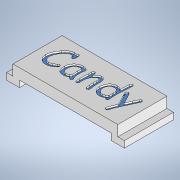
# Autodesk Inventor part: Крышка аккумулятора
Saved by Autodesk Inventor 2020 (Build 240168000, 168)
## iProperties
Created: 2021-04-26
Part Number: Крышка аккумулятора
Material: Типовые
Document SubType Name: Обычные детали
Designer: Антон
Density: 1 g/cm^3
Appearance: Белый
Sheet Metal Rule: По умолчанию
Author: Антон
Autodesk Inventor part; units mm, degrees
ref_plane "YZ Plane" through (0, 0, 0) normal (1, 0, 0) x (0, 1, 0)
ref_plane "XZ Plane" through (0, 0, 0) normal (0, 1, 0) x (-1, 0, 0)
ref_plane "XY Plane" through (0, 0, 0) normal (0, 0, 1) x (1, 0, 0)
sketch "Эскиз1" plane through (0, 0, 0) normal (0, 0, 1) x (1, 0, 0)
  line L0 (0, 0) -> (32, 0)
  line L1 (32, 0) -> (32, 5.25)
  line L2 (32, 5.25) -> (0, 5.25)
  line L3 (0, 5.25) -> (0, 0)
  line L4 (32, 2) -> (34, 2)
  line L5 (34, 2) -> (34, 0)
  line L6 (34, 0) -> (32, 0)
  line L7 (32, 0) -> (32, 2)
  line L8 (-2, 0) -> (0, 0)
  line L9 (0, 0) -> (0, 2)
  line L10 (0, 2) -> (-2, 2)
  line L11 (-2, 2) -> (-2, 0)
  point P0 (0, 2)
  dimension "d32" = 32
  dimension "d33" = 5.25
  dimension "d34" = 2
  dimension "d35" = 2
  constraints: 24 end point, 6 parallel, 4 collinear, 3 horizontal, 3 perpendicular, 2 equal length
  measures "d32" distance of L2.end L1.end
  measures "d33" distance of L1.end L0.end
  measures "d34" distance of L5.end L6.end
  measures "d35" distance of L4.end L5.end
extrude "Выдавливание1" add sketch "Эскиз1" along normal blind 15
sketch "Эскиз9" plane through (0, 0, 15) normal (0, 0, 1) x (1, 0, 0)
  line L0 (0, 5.25) -> (0, 2) projected
  line L1 (32, 5.25) -> (0, 5.25) projected
  line L2 (0, 2) -> (32, 2)
  line L3 (32, 2) -> (32, 5.25)
  line L4 (32, 5.25) -> (0, 5.25)
  line L5 (0, 5.25) -> (0, 2)
  line L6 (-2, 0) -> (34, 0) projected
  line L7 (0, 2) -> (2, 2)
  line L8 (2, 2) -> (2, 0)
  line L9 (2, 0) -> (0, 0)
  line L10 (0, 0) -> (0, 2)
  line L11 (32, 2) -> (32, 5.25) projected
  line L12 (32, 2) -> (30, 2)
  line L13 (30, 2) -> (30, 0)
  line L14 (30, 0) -> (32, 0)
  line L15 (32, 0) -> (32, 2)
  line L16 (34, 2) -> (32, 2) projected
  line L17 (0, 2) -> (-2, 2) projected
  constraints: 24 end point, 6 parallel, 3 horizontal, 3 perpendicular, 2 collinear, 2 point on line
extrude "Выдавливание9" cut sketch "Эскиз9" against normal blind 14 contours L2 L13 L6 L8
sketch "Эскиз8" plane through (0, 5.25, 0) normal (0, 1, 0) x (1, 0, 0)
  line L0 (0, 0) -> (32, 0) construction
  line L1 (32, 0) -> (32, -15) construction
  line L2 (32, -15) -> (0, -15) construction
  line L3 (0, -15) -> (0, 0) construction
  spline S0 degree 2 poles (7.5517, -4.4655) (7.2345, -4.4655) (7.0759, -4.0931) knots 0 0 0 1 1 1
  spline S1 degree 2 poles (7.0759, -4.0931) (6.9379, -3.7759) (6.8207, -3.7069) knots 0 0 0 1 1 1
  spline S2 degree 2 poles (6.8207, -3.7069) (6.7172, -3.6517) (6.3034, -3.6517) knots 0 0 0 1 1 1
  spline S3 degree 2 poles (6.3034, -3.6517) (5.5862, -3.6517) (4.7103, -4.7483) knots 0 0 0 1 1 1
  spline S4 degree 2 poles (4.7103, -4.7483) (3.5241, -6.2241) (3.5241, -7.5414) knots 0 0 0 1 1 1
  spline S5 degree 2 poles (3.5241, -7.5414) (3.5241, -8.1828) (3.9379, -8.6379) knots 0 0 0 1 1 1
  spline S6 degree 2 poles (3.9379, -8.6379) (4.3586, -9.1138) (4.9517, -9.1138) knots 0 0 0 1 1 1
  spline S7 degree 2 poles (4.9517, -9.1138) (5.4621, -9.1138) (5.9724, -8.8517) knots 0 0 0 1 1 1
  spline S8 degree 2 poles (5.9724, -8.8517) (6.2621, -8.7) (6.8552, -8.2655) knots 0 0 0 1 1 1
  spline S9 degree 2 poles (6.8552, -8.2655) (7.1379, -8.0586) (7.2828, -8.0586) knots 0 0 0 1 1 1
  spline S10 degree 2 poles (7.2828, -8.0586) (7.4897, -8.0586) (7.7793, -8.3828) (7.7793, -8.5759) knots 0 0 0 1 2 2 2
  spline S11 degree 2 poles (7.7793, -8.5759) (7.7793, -8.8034) (7.5931, -8.969) knots 0 0 0 1 1 1
  spline S12 degree 2 poles (7.5931, -8.969) (6.2828, -10.1276) (4.9517, -10.1276) knots 0 0 0 1 1 1
  spline S13 degree 2 poles (4.9517, -10.1276) (3.9241, -10.1276) (3.2207, -9.3414) knots 0 0 0 1 1 1
  spline S14 degree 2 poles (3.2207, -9.3414) (2.5379, -8.5828) (2.5379, -7.5414) knots 0 0 0 1 1 1
  spline S15 degree 2 poles (2.5379, -7.5414) (2.5379, -5.8655) (3.9448, -4.1069) knots 0 0 0 1 1 1
  spline S16 degree 2 poles (3.9448, -4.1069) (5.1172, -2.6379) (6.3034, -2.6379) knots 0 0 0 1 1 1
  spline S17 degree 2 poles (6.3034, -2.6379) (6.5448, -2.6379) (6.931, -2.6793) (7.0828, -2.7345) knots 0 0 0 1 2 2 2
  spline S18 degree 2 poles (7.0828, -2.7345) (7.2552, -2.4793) (7.531, -2.4793) knots 0 0 0 1 1 1
  spline S19 degree 2 poles (7.531, -2.4793) (7.8759, -2.4793) (7.9655, -2.9276) knots 0 0 0 1 1 1
  spline S20 degree 2 poles (7.9655, -2.9276) (8.0414, -3.3345) (8.0414, -3.9138) knots 0 0 0 1 1 1
  spline S21 degree 2 poles (8.0414, -3.9138) (8.0414, -4.1207) (7.931, -4.2724) knots 0 0 0 1 1 1
  spline S22 degree 2 poles (7.931, -4.2724) (7.8, -4.4655) (7.5517, -4.4655) knots 0 0 0 1 1 1
  spline S23 degree 2 poles (12.7448, -10.3414) (12.6552, -10.3414) (12.4069, -10.1207) knots 0 0 0 1 1 1
  spline S24 degree 2 poles (12.4069, -10.1207) (12.1862, -9.9207) (12.0759, -9.7621) knots 0 0 0 1 1 1
  spline S25 degree 2 poles (12.0759, -9.7621) (11.6, -10.0172) (10.8759, -10.2793) (10.6345, -10.2793) knots 0 0 0 1 2 2 2
  spline S26 degree 2 poles (10.6345, -10.2793) (9.4759, -10.2793) (8.9448, -9.6241) knots 0 0 0 1 1 1
  spline S27 degree 2 poles (8.9448, -9.6241) (8.4483, -9.0103) (8.4483, -7.7483) knots 0 0 0 1 1 1
  spline S28 degree 2 poles (8.4483, -7.7483) (8.4483, -6.5483) (10.0966, -4.8448) (11.2414, -4.8448) knots 0 0 0 1 2 2 2
  spline S29 degree 2 poles (11.2414, -4.8448) (11.669, -4.8448) (12.2069, -5.0655) knots 0 0 0 1 1 1
  spline S30 degree 2 poles (12.2069, -5.0655) (12.8759, -5.3483) (12.8759, -5.7345) knots 0 0 0 1 1 1
  spline S31 degree 2 poles (12.8759, -5.7345) (12.8759, -5.8724) (12.7793, -5.9759) knots 0 0 0 1 1 1
  spline S32 degree 2 poles (12.7793, -5.9759) (12.731, -6.1621) (12.6759, -7.0241) (12.669, -7.7) knots 0 0 0 1 2 2 2
  spline S33 degree 2 poles (12.669, -7.7) (12.6621, -8.3138) (12.7517, -8.6655) knots 0 0 0 1 1 1
  spline S34 degree 2 poles (12.7517, -8.6655) (12.8, -8.8862) (13.0621, -9.5414) knots 0 0 0 1 1 1
  spline S35 degree 2 poles (13.0621, -9.5414) (13.0966, -9.631) (13.1793, -9.8034) knots 0 0 0 1 1 1
  line L4 (13.1793, -9.8034) -> (13.2069, -9.8862)
  spline S36 degree 2 poles (13.2069, -9.8862) (13.2069, -10.0862) (12.931, -10.3414) (12.7448, -10.3414) knots 0 0 0 1 2 2 2
  spline S37 degree 2 poles (11.7172, -6.9) (11.7172, -6.6862) (11.7724, -6.1828) (11.8276, -5.9069) knots 0 0 0 1 2 2 2
  spline S38 degree 2 poles (11.8276, -5.9069) (11.6414, -5.8103) (11.3793, -5.7207) (11.3034, -5.7207) knots 0 0 0 1 2 2 2
  spline S39 degree 2 poles (11.3034, -5.7207) (10.531, -5.7207) (9.4207, -6.969) (9.4207, -7.7897) knots 0 0 0 1 2 2 2
  spline S40 degree 2 poles (9.4207, -7.7897) (9.4207, -8.5966) (9.9931, -9.4103) (10.5724, -9.4103) knots 0 0 0 1 2 2 2
  spline S41 degree 2 poles (10.5724, -9.4103) (11.0414, -9.4103) (11.3724, -9.2379) knots 0 0 0 1 1 1
  spline S42 degree 2 poles (11.3724, -9.2379) (11.5517, -9.1414) (11.8759, -8.8586) knots 0 0 0 1 1 1
  spline S43 degree 2 poles (11.8759, -8.8586) (11.7172, -7.5483) (11.7172, -6.9) knots 0 0 0 1 1 1
  spline S44 degree 2 poles (17.8621, -10.3621) (17.4414, -10.3621) (17.3862, -9.9) knots 0 0 0 1 1 1
  line L5 (17.3862, -9.9) -> (17.2483, -8.8103)
  spline S45 degree 2 poles (17.2483, -8.8103) (17.1793, -8.231) (17.1793, -7.7276) knots 0 0 0 1 1 1
  spline S46 degree 2 poles (17.1793, -7.7276) (17.1793, -7.5897) (17.2138, -6.9276) (17.2138, -6.7897) knots 0 0 0 1 2 2 2
  spline S47 degree 2 poles (17.2138, -6.7897) (17.2138, -5.7207) (16.8207, -5.7207) knots 0 0 0 1 1 1
  spline S48 degree 2 poles (16.8207, -5.7207) (16.2621, -5.7207) (15.7586, -6.3759) knots 0 0 0 1 1 1
  spline S49 degree 2 poles (15.7586, -6.3759) (15.3034, -6.9759) (15.0483, -7.8931) knots 0 0 0 1 1 1
  spline S50 degree 2 poles (15.0483, -7.8931) (15.0345, -8.0862) (15, -8.3759) knots 0 0 0 1 1 1
  spline S51 degree 2 poles (15, -8.3759) (14.9724, -8.6241) (14.9724, -8.8586) knots 0 0 0 1 1 1
  spline S52 degree 2 poles (14.9724, -8.8586) (14.9724, -9.0034) (15.0345, -9.5966) (15.0345, -9.7483) knots 0 0 0 1 2 2 2
  spline S53 degree 2 poles (15.0345, -9.7483) (15.0345, -9.969) (14.7586, -10.2448) (14.5448, -10.2448) knots 0 0 0 1 2 2 2
  spline S54 degree 2 poles (14.5448, -10.2448) (14.331, -10.2448) (14.0621, -9.969) (14.0621, -9.7483) knots 0 0 0 1 2 2 2
  spline S55 degree 2 poles (14.0621, -9.7483) (14.0621, -9.5966) (14, -9.0034) (14, -8.8517) knots 0 0 0 1 2 2 2
  spline S56 degree 2 poles (14, -8.8517) (14, -8.3414) (14.1379, -6.5414) (14.1379, -6.031) knots 0 0 0 1 2 2 2
  spline S57 degree 2 poles (14.1379, -6.031) (14.1379, -5.8724) (14.1034, -5.2448) (14.1034, -5.0862) knots 0 0 0 1 2 2 2
  spline S58 degree 2 poles (14.1034, -5.0862) (14.1034, -4.8724) (14.3862, -4.6034) (14.5931, -4.6034) knots 0 0 0 1 2 2 2
  spline S59 degree 2 poles (14.5931, -4.6034) (15.0483, -4.6034) (15.0966, -5.2517) knots 0 0 0 1 1 1
  line L6 (15.0966, -5.2517) -> (15.1103, -5.831)
  spline S60 degree 2 poles (15.1103, -5.831) (15.9379, -4.7207) (16.8138, -4.7207) knots 0 0 0 1 1 1
  spline S61 degree 2 poles (16.8138, -4.7207) (17.6069, -4.7207) (17.9172, -5.4172) knots 0 0 0 1 1 1
  spline S62 degree 2 poles (17.9172, -5.4172) (18.131, -5.8862) (18.1517, -6.7966) knots 0 0 0 1 1 1
  line L7 (18.1517, -6.7966) -> (18.1517, -7.2931)
  line L8 (18.1517, -7.2931) -> (18.1448, -7.7552)
  spline S63 degree 2 poles (18.1448, -7.7552) (18.1448, -8.1621) (18.3586, -9.4655) (18.3586, -9.8724) knots 0 0 0 1 2 2 2
  spline S64 degree 2 poles (18.3586, -9.8724) (18.3586, -10.0931) (18.0759, -10.3621) (17.8621, -10.3621) knots 0 0 0 1 2 2 2
  spline S65 degree 2 poles (23.931, -5.6448) (23.869, -6.369) (23.869, -7.1) knots 0 0 0 1 1 1
  spline S66 degree 2 poles (23.869, -7.1) (23.869, -8.7483) (24.0207, -9.5897) knots 0 0 0 1 1 1
  spline S67 degree 2 poles (24.0207, -9.5897) (24.0345, -9.6586) (24.0345, -9.7) knots 0 0 0 1 1 1
  spline S68 degree 2 poles (24.0345, -9.7) (24.0345, -9.9) (23.7586, -10.1552) (23.5724, -10.1552) knots 0 0 0 1 2 2 2
  spline S69 degree 2 poles (23.5724, -10.1552) (23.269, -10.1552) (23.1241, -9.7069) knots 0 0 0 1 1 1
  spline S70 degree 2 poles (23.1241, -9.7069) (22.7655, -9.969) (22, -10.2379) (21.5862, -10.2379) knots 0 0 0 1 2 2 2
  spline S71 degree 2 poles (21.5862, -10.2379) (20.5586, -10.2379) (19.8897, -9.5552) knots 0 0 0 1 1 1
  spline S72 degree 2 poles (19.8897, -9.5552) (19.1931, -8.8586) (19.1931, -7.7621) knots 0 0 0 1 1 1
  spline S73 degree 2 poles (19.1931, -7.7621) (19.1931, -6.4448) (20.5931, -4.8517) (21.7103, -4.8517) knots 0 0 0 1 2 2 2
  spline S74 degree 2 poles (21.7103, -4.8517) (22.2828, -4.8517) (22.6, -5.031) knots 0 0 0 1 1 1
  line L9 (22.6, -5.031) -> (23.0621, -5.369)
  spline S75 degree 2 poles (23.0621, -5.369) (23.131, -3.2862) (23.2276, -2.569) knots 0 0 0 1 1 1
  spline S76 degree 2 poles (23.2276, -2.569) (23.2897, -2.1276) (23.6759, -2.1276) knots 0 0 0 1 1 1
  spline S77 degree 2 poles (23.6759, -2.1276) (24.1241, -2.1276) (24.1241, -2.6103) knots 0 0 0 1 1 1
  spline S78 degree 2 poles (24.1241, -2.6103) (24.1241, -3.2931) (23.931, -5.6448) knots 0 0 0 1 1 1
  spline S79 degree 2 poles (21.731, -5.769) (20.9034, -5.769) (20.069, -6.7552) (20.069, -7.7414) knots 0 0 0 1 2 2 2
  spline S80 degree 2 poles (20.069, -7.7414) (20.069, -8.3828) (20.9724, -9.3) (21.5862, -9.3) knots 0 0 0 1 2 2 2
  spline S81 degree 2 poles (21.5862, -9.3) (22, -9.3) (22.2897, -9.1483) knots 0 0 0 1 1 1
  spline S82 degree 2 poles (22.2897, -9.1483) (22.4552, -9.0586) (22.8345, -8.7345) knots 0 0 0 1 1 1
  spline S83 degree 2 poles (22.8345, -8.7345) (22.9103, -8.6724) (22.9793, -8.5828) knots 0 0 0 1 1 1
  line L10 (22.9793, -8.5828) -> (22.9655, -7.7276)
  line L11 (22.9655, -7.7276) -> (22.9724, -7.1552)
  line L12 (22.9724, -7.1552) -> (22.9793, -6.569)
  spline S84 degree 2 poles (22.9793, -6.569) (22.7931, -6.169) (22.1655, -5.769) (21.731, -5.769) knots 0 0 0 1 2 2 2
  line L13 (29.6345, -5.5966) -> (27.9241, -9.3)
  spline S85 degree 2 poles (27.9241, -9.3) (27.2897, -10.6517) (26.9517, -11.5621) knots 0 0 0 1 1 1
  line L14 (26.9517, -11.5621) -> (26.6276, -12.5207)
  spline S86 degree 2 poles (26.6276, -12.5207) (26.4966, -12.8724) (26.1862, -12.8724) knots 0 0 0 1 1 1
  spline S87 degree 2 poles (26.1862, -12.8724) (25.9793, -12.8724) (25.6759, -12.6034) (25.6759, -12.3966) knots 0 0 0 1 2 2 2
  spline S88 degree 2 poles (25.6759, -12.3966) (25.6759, -11.9069) (26.7448, -9.5345) knots 0 0 0 1 1 1
  line L15 (26.7448, -9.5345) -> (24.9724, -6.1276)
  line L16 (24.9724, -6.1276) -> (24.7448, -5.769)
  spline S89 degree 2 poles (24.7448, -5.769) (24.6138, -5.5414) (24.6138, -5.3828) knots 0 0 0 1 1 1
  spline S90 degree 2 poles (24.6138, -5.3828) (24.6138, -5.1828) (24.9241, -4.8724) (25.1172, -4.8724) knots 0 0 0 1 2 2 2
  spline S91 degree 2 poles (25.1172, -4.8724) (25.3448, -4.8724) (25.469, -5.0517) knots 0 0 0 1 1 1
  spline S92 degree 2 poles (25.469, -5.0517) (26.3103, -6.2241) (27.2759, -8.3897) knots 0 0 0 1 1 1
  line L17 (27.2759, -8.3897) -> (28.0138, -6.6655)
  spline S93 degree 2 poles (28.0138, -6.6655) (28.4069, -5.7828) (28.7724, -5.1414) knots 0 0 0 1 1 1
  spline S94 degree 2 poles (28.7724, -5.1414) (28.931, -4.8655) (29.1862, -4.8655) knots 0 0 0 1 1 1
  spline S95 degree 2 poles (29.1862, -4.8655) (29.3862, -4.8655) (29.6966, -5.1552) (29.6966, -5.3483) knots 0 0 0 1 2 2 2
  spline S96 degree 2 poles (29.6966, -5.3483) (29.6966, -5.4586) (29.6345, -5.5966) knots 0 0 0 1 1 1
  constraints: 3 coincident, 2 other
emboss "Рельеф1" sketch "Эскиз8" operation cut depth 0.5 direction (0, -1, 0)
equation "\"Радиус_гибки\" = Толщина"
equation "\"Ширина_просечки\" = Толщина"
equation "\"Глубина_просечки\" = 0.5 * Толщина"
equation "\"Размер_просечки\" = 4 * Толщина"
equation "\"Мин_остаток\" = 2 * Толщина"
equation "\"Радиус_перехода\" = Радиус_гибки"
equation "\"Радиус_Якоби\" = Толщина"
equation "\"Размер_зазора\" = Толщина"
equation "\"Толщина\" = 0.5"
